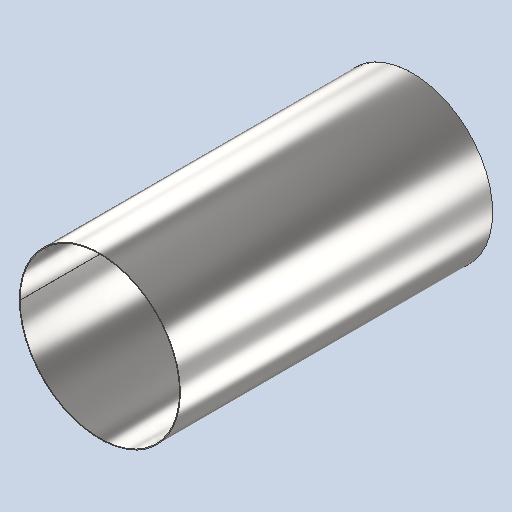
# Autodesk Inventor part: MSC 082 rocket body
Saved by Autodesk Inventor 2024.2 (Build 282272000, 272)
## iProperties
Created: 2024-05-19
Part Number: MSC 082 rocket body
Material: Stainless Steel
Document SubType Name: Sheet Metal
Designer: admin
Density: 8 g/cm^3
Flat Pattern Width: 32 cm
Flat Pattern Length: 51.5405 cm
Flat Pattern Area: 1649.3 cm^2
Sheet Metal Rule: Default
Sheet Metal Width: 320,000 mm
Sheet Metal Length: 515,405 mm
Sheet Metal Area: 164929,508 mm^2
Appearance: Semi-Polished
Stock Number: МОО 082 ракета тело
Author: admin
Autodesk Inventor part; units mm, degrees
ref_plane "YZ Plane" through (0, 0, 0) normal (1, 0, 0) x (0, 1, 0)
ref_plane "XZ Plane" through (0, 0, 0) normal (0, 1, 0) x (-1, 0, 0)
ref_plane "XY Plane" through (0, 0, 0) normal (0, 0, 1) x (1, 0, 0)
sketch "Sketch1" plane through (0, 0, 0) normal (0, 0, 1) x (1, 0, 0)
  line L0 (0, 0) -> (0, 320)
  line L1 (-81.7, 320) -> (-82.5, 320)
  line L2 (-82.5, 320) -> (-82.5, 0)
  line L3 (-82.5, 0) -> (-81.7, 0)
  line L4 (-81.7, 0) -> (-81.7, 320)
  line L5 (-81.7, 320) -> (-82.5, 0) construction
  line L6 (-82.5, 320) -> (-81.7, 0) construction
  point P0 (-82.1, 160)
  dimension "d0" = 320
  dimension "d1" = 0.8
  dimension "d2" = 165
  constraints: 14 end point, 2 midpoint, 2 parallel, 2 point on line, 1 horizontal, 1 perpendicular, 1 vertical
  measures "d0" distance of L0.start L0.end
  measures "d1" distance of L1.start L1.end
  measures "d2" diameter of L2 L0
revolve "Revolution1" add sketch "Sketch1" angle 359.9 about axis through (0, 0, 0) along (0, 1, 0)
equation "\"d1\" = Thickness"
equation "\"BendRadius\" = Thickness"
equation "\"BendReliefWidth\" = Thickness"
equation "\"BendReliefDepth\" = 0.5 * Thickness"
equation "\"CornerReliefSize\" = 4 * Thickness"
equation "\"MinimumRemnant\" = 2 * Thickness"
equation "\"TransitionRadius\" = BendRadius"
equation "\"JacobiRadiusSize\" = BendRadius"
equation "\"GapSize\" = Thickness"
equation "\"Thickness\" = 0.8"
body "Solid1"
